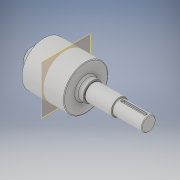
# Autodesk Inventor part: vratilo
Saved by Autodesk Inventor 2018 (Build 220112000, 112)
## iProperties
Created: 2018-05-05
Part Number: vratilo
Material: Generic
Document SubType Name: Modeling
Designer: Kristijan
Density: 1 g/cm^3
Appearance: Default
Author: Kristijan
Autodesk Inventor part; units mm, degrees
ref_plane "YZ Plane" through (0, 0, 0) normal (1, 0, 0) x (0, 1, 0)
ref_plane "XZ Plane" through (0, 0, 0) normal (0, 1, 0) x (-1, 0, 0)
sketch "Sketch1" plane through (0, 0, 0) normal (1, 0, 0) x (0, 1, 0)
  circle A0 centre (0, 0) radius 60.5
  dimension "d0" = 121
  constraints: 1 centre point, 1 coincident
  measures "d0" diameter of A0
extrude "Extrusion1" add sketch "Sketch1" along normal mid plane 115
sketch "Sketch2" plane through (57.5, 0, 0) normal (1, 0, 0) x (0, 0, -1)
  circle A0 centre (0, 0) radius 26
  dimension "d3" = 52
  constraints: 1 centre point, 1 coincident
  measures "d3" diameter of A0
extrude "Extrusion2" add sketch "Sketch2" along normal blind 18
sketch "Sketch3" plane through (75.5, 0, 0) normal (1, 0, 0) x (0, 0, -1)
  circle A0 centre (0, 0) radius 22.5
  dimension "d6" = 45
  constraints: 1 centre point, 1 coincident
  measures "d6" diameter of A0
extrude "Extrusion3" add sketch "Sketch3" along normal blind 73
sketch "Sketch4" plane through (148.5, 0, 0) normal (1, 0, 0) x (0, 0, -1)
  circle A0 centre (0, 0) radius 19
  dimension "d9" = 38
  constraints: 1 centre point, 1 coincident
  measures "d9" diameter of A0
extrude "Extrusion4" add sketch "Sketch4" along normal blind 80
sketch "Sketch9" plane through (-57.5, 0, 0) normal (-1, 0, 0) x (0, 0, 1)
  point P0 (0, 0)
sketch "Sketch10" plane through (-57.5, 0, 0) normal (-1, 0, 0) x (0, 0, 1)
  circle A0 centre (0, 0) radius 26
  dimension "d45" = 52
  constraints: 1 centre point, 1 coincident
  measures "d45" diameter of A0
extrude "Extrusion8" add sketch "Sketch10" along normal blind 13
sketch "Sketch11" plane through (-70.5, 0, 0) normal (-1, 0, 0) x (0, 0, 1)
  circle A0 centre (0, 0) radius 22.5
  dimension "d48" = 45
  constraints: 1 centre point, 1 coincident
  measures "d48" diameter of A0
extrude "Extrusion9" add sketch "Sketch11" along normal blind 21
ref_plane "Work Plane1" through (148.5, 0, 19) normal (0, 0, 1) x (1, 0, 0)
sketch "Sketch6" plane through (148.5, 0, 19) normal (0, 0, 1) x (1, 0, 0)
  line L0 (9, 0) -> (71, 0) construction
  line L1 (9, -4) -> (71, -4)
  line L2 (71, 4) -> (9, 4)
  arc A0 (9, 4) -> (9, -4) centre (9, 0) ccw
  arc A1 (71, -4) -> (71, 4) centre (71, 0) ccw
  line L3 (80, -19) -> (80, 19) construction
  line L4 (-263.2, 0) -> (137.2, 0) construction
  line L5 (0, -22.5) -> (0, 22.5) construction
  point P0 (-148.5, 0)
  point P1 (40, 0)
  dimension "d15" = 62
  dimension "d16" = 8
  dimension "d18" = 5
  constraints: 8 end point, 4 point on circle, 4 tangent, 2 centre point, 1 collinear, 1 horizontal, 1 midpoint, 1 parallel
  measures "d15" distance of L0.start L0.end
  measures "d16" diameter of A1
  measures "d18" distance edge to line of A1 L3
extrude "Extrusion6" cut sketch "Sketch6" against normal blind 5
sketch "Sketch7" plane through (0, 0, 0) normal (0, 1, 0) x (-1, 0, 0)
  line L0 (-57.5, -26) -> (-75.5, -26) construction
  line L1 (-75.5, -26) -> (-75.5, -22.5) construction
  line L2 (-75.5, -22.5) -> (-148.5, -22.5) construction
  line L3 (-148.5, -22.5) -> (-148.5, -19) construction
  line L4 (-148.5, -19) -> (-228.5, -19) construction
  line L5 (-228.5, -19) -> (-228.5, 19) construction
  line L6 (-228.5, 19) -> (-223.5, 19) construction
  line L7 (-223.5, 19) -> (-223.5, 14) construction
  line L8 (-223.5, 14) -> (-153.5, 14) construction
  line L9 (-153.5, 14) -> (-153.5, 19) construction
  line L10 (-153.5, 19) -> (-148.5, 19) construction
  line L11 (-148.5, 19) -> (-148.5, 22.5) construction
  line L12 (-148.5, 22.5) -> (-75.5, 22.5) construction
  line L13 (-75.5, 22.5) -> (-75.5, 26) construction
  line L14 (-75.5, 26) -> (-57.5, 26) construction
  line L15 (-57.5, 26) -> (-57.5, 60.5) construction
  line L16 (-57.5, 60.5) -> (57.5, 60.5) construction
  line L17 (57.5, 60.5) -> (57.5, 26) construction
  line L18 (57.5, -60.5) -> (-57.5, -60.5) construction
  line L19 (-57.5, -60.5) -> (-57.5, -26) construction
  line L20 (-78, 15.4374) -> (-78, 22.5) construction
  line L21 (-75.5, 22.5) -> (-148.5, 22.5) construction
  line L22 (-78, 22.5) -> (-75.5, 22.5)
  line L23 (-75.5, 22.2) -> (-76.8804, 22.2)
  line L24 (-75.5, 26) -> (-75.5, -26) construction
  line L25 (-78, 22.5) -> (-76.8804, 22.2)
  line L26 (-75.5, 22.5) -> (-78, 22.5) construction
  line L27 (-75.5, 22.5) -> (-75.5, 22.2)
  line L28 (125.9, 0) -> (-198.9, 0) projected
  line L29 (57.5, 26) -> (70.5, 26) projected
  line L30 (70.5, 26) -> (70.5, 22.5) projected
  line L31 (70.5, 22.5) -> (91.5, 22.5) projected
  line L32 (91.5, 22.5) -> (91.5, -22.5) projected
  line L33 (91.5, -22.5) -> (70.5, -22.5) projected
  line L34 (70.5, -22.5) -> (70.5, -26) projected
  line L35 (70.5, -26) -> (57.5, -26) projected
  line L36 (57.5, -26) -> (57.5, -60.5) projected
  point P0 (0, 0)
  dimension "d21" = 2.5
  dimension "d24" = 0.3
  dimension "d25" = 15
  constraints: 12 end point, 3 point on line, 2 collinear, 2 horizontal, 1 vertical
  measures "d21" distance between parallel lines of L20 L13
  measures "d24" distance between parallel lines of L12 L23
  measures "d25" angle of L12 L25
revolve "Revolution1" cut sketch "Sketch7" angle 360 about axis through (-10, 0, 0) along (1, 0, 0)
ref_plane "Work Plane2" through (2.5, 0, 0) normal (1, 0, 0) x (0, 0, -1)
mirror "Mirror3" about plane through (2.5, 0, 0) normal (1, 0, 0) of "Revolution1"
fillet "Fillet1" radius 0.6 2 edges at (75.5, 0, -22.2) (-70.5, 0, -22.2)
fillet "Fillet2" radius 0.6 1 edges at (76.8804, 0, -22.2)
fillet "Fillet5" radius 1 1 edges at (148.5, 0, 19)
fillet "Fillet6" radius 5 2 edges at (57.5, 0, 26) (-57.5, 0, -26)
chamfer "Chamfer1" distance 1.5 angle 45 2 edges at (228.5, 0, 19) (-91.5, 0, -22.5)
chamfer "Chamfer2" distance 2 angle 30 1 edges at (57.5, -60.5, 0) measured on face at (57.5, -60, 0)
chamfer "Chamfer3" distance 2 angle 30 1 edges at (-57.5, -60.5, 0) measured on face at (-57.5, -60, 0)
body "Solid1"
